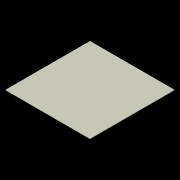
# Autodesk Inventor part: PolyBase
Saved by Autodesk Inventor 2016 (Build 200138000, 138)
## iProperties
Created: 2017-01-21
Part Number: PolyBase
Material: UHMW, White
Document SubType Name: Modeling
Designer: Alexis Renderos
Density: 0.94 g/cm^3
Appearance: Ivory Flat
Author: Alexis Renderos
Autodesk Inventor part; units mm, degrees
ref_plane "YZ Plane" through (0, 0, 0) normal (1, 0, 0) x (0, 1, 0)
ref_plane "XZ Plane" through (0, 0, 0) normal (0, 1, 0) x (-1, 0, 0)
ref_plane "XY Plane" through (0, 0, 0) normal (0, 0, 1) x (1, 0, 0)
sketch "Sketch1" plane through (0, 0, 0) normal (0, 1, 0) x (-1, 0, 0)
  line L0 (0, -640.08) -> (0, 640.08) projected
  line L1 (-640.08, 0) -> (640.08, 0) projected
  line L2 (457.2, 457.2) -> (-457.2, 457.2)
  line L3 (-457.2, 457.2) -> (-457.2, -457.2)
  line L4 (-457.2, -457.2) -> (457.2, -457.2)
  line L5 (457.2, -457.2) -> (457.2, 457.2)
  point P0 (0, 0)
  dimension "d0" = 914.4
  dimension "d1" = 914.4
  constraints: 8 end point, 2 parallel, 1 horizontal, 1 perpendicular, 2 other
  measures "d0" distance of L4.end L3.end
  measures "d1" distance of L3.end L2.end
extrude "Extrusion1" add sketch "Sketch1" along normal blind 6.35
body "Solid1"
